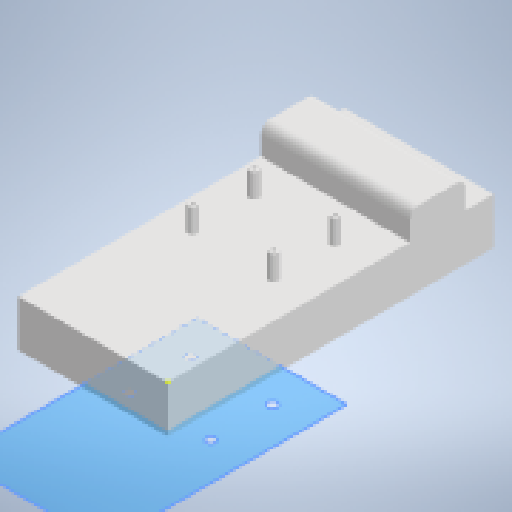
# Autodesk Inventor part: CarApproximation
Saved by Autodesk Inventor 2024.2 (Build 282272000, 272)
## iProperties
Created: 2024-04-01
Part Number: CarApproximation
Material: Generic
Document SubType Name: Modeling
Designer: ringl
Density: 1 g/cm^3
Appearance: Default
Author: ringl
Autodesk Inventor part; units mm, degrees
ref_plane "YZ Plane" through (0, 0, 0) normal (1, 0, 0) x (0, 1, 0)
ref_plane "XZ Plane" through (0, 0, 0) normal (0, 1, 0) x (-1, 0, 0)
ref_plane "XY Plane" through (0, 0, 0) normal (0, 0, 1) x (1, 0, 0)
sketch "Sketch1" plane through (0, 0, 0) normal (0, 1, 0) x (-1, 0, 0)
  line L0 (0, 0) -> (80, 0)
  line L1 (80, 0) -> (80, -175)
  line L2 (80, -175) -> (0, -175)
  line L3 (0, -175) -> (0, 0)
  dimension "d0" = 80
  dimension "d1" = 175
  constraints: 8 end point, 2 parallel, 1 horizontal, 1 perpendicular
  measures "d0" distance of L1.end L2.end
  measures "d1" distance of L0.end L1.end
extrude "Extrusion1" add sketch "Sketch1" along normal blind 25
sketch "Sketch2" plane through (0, 25, 0) normal (0, 1, 0) x (1, 0, 0)
  point P0 (0, 0)
sketch "Sketch3" plane through (0, 0, 0) normal (1, 0, 0) x (0, 0, -1)
  line L0 (175, 25) -> (0, 25) projected
  line L1 (160, 25) -> (130, 25)
  line L2 (130, 25) -> (130, 40)
  line L3 (130, 40) -> (160, 40)
  line L4 (160, 40) -> (160, 25)
  line L5 (175, 0) -> (175, 25) projected
  point P0 (0, 0)
  dimension "d4" = 15
  dimension "d5" = 15
  dimension "d6" = 30
  constraints: 8 end point, 2 parallel, 1 horizontal, 1 perpendicular, 1 point on line
  measures "d4" distance between parallel lines of L5 L4
  measures "d5" distance of L3.end L1.start
  measures "d6" distance of L2.end L3.end
extrude "Extrusion2" add sketch "Sketch3" against normal blind 80
fillet "Fillet1" radius 5 2 edges at (-40, 40, -130) (-40, 40, -160)
sketch "Sketch4" plane through (0, 25, 0) normal (0, 1, 0) x (1, 0, 0)
  circle A0 centre (-63.5, 110) radius 2.5
  circle A1 centre (-20, 110) radius 2.5
  circle A2 centre (-20, 77) radius 2.5
  circle A3 centre (-63.5, 77) radius 2.5
  line L0 (0, 0) -> (0, 130) projected
  line L1 (-80, 130) -> (0, 130) projected
  dimension "d10" = 5
  dimension "d11" = 5
  dimension "d12" = 5
  dimension "d13" = 5
  dimension "d14" = 20
  dimension "d15" = 20
  dimension "d16" = 43.5
  dimension "d17" = 43.5
  dimension "d18" = 20
  dimension "d19" = 20
  dimension "d20" = 33
  dimension "d21" = 33
  constraints: 4 centre point
  measures "d10" diameter of A0
  measures "d11" diameter of A1
  measures "d12" diameter of A2
  measures "d13" diameter of A3
  measures "d14" distance from line of L0 A1.centre
  measures "d15" distance from line of L0 A2.centre
  measures "d16" distance of A1.centre A0.centre
  measures "d17" distance of A2.centre A3.centre
  measures "d18" distance from line of A0.centre L1
  measures "d19" distance from line of A1.centre L1
  measures "d20" distance of A2.centre A1.centre
  measures "d21" distance of A0.centre A3.centre
extrude "Extrusion3" add sketch "Sketch4" along normal blind 13
sketch "Sketch5" plane through (-20, 38, -77) normal (0, 1, 0) x (1, 0, 0)
  circle A0 centre (-43.5, 0) radius 2.5 projected
  circle A1 centre (-43.5, 0) radius 1
  circle A2 centre (-43.5, 33) radius 2.5 projected
  circle A3 centre (-43.5, 33) radius 1
  circle A4 centre (0, 33) radius 2.5 projected
  circle A5 centre (0, 33) radius 1
  circle A6 centre (0, 0) radius 2.5 projected
  circle A7 centre (0, 0) radius 1
  point P0 (20, -77)
  dimension "d24" = 2
  dimension "d25" = 2
  dimension "d26" = 2
  dimension "d27" = 2
  constraints: 4 centre point, 4 coincident
  measures "d24" diameter of A1
  measures "d25" diameter of A3
  measures "d26" diameter of A5
  measures "d27" diameter of A7
extrude "Extrusion4" cut sketch "Sketch5" against normal blind 13 contours A1 | A3 | A5 | A7
body "Solid1"
